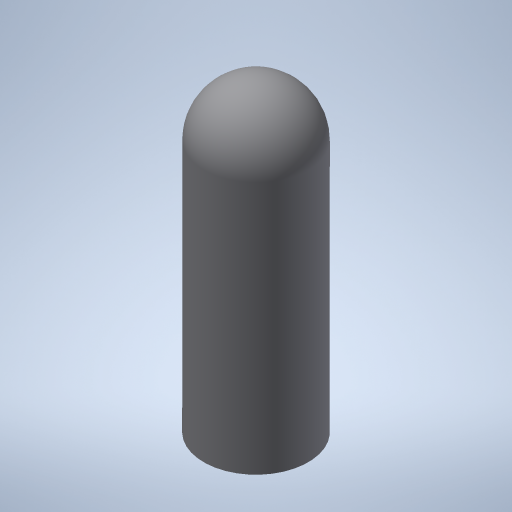
# Autodesk Inventor part: continuacion medio
Saved by Autodesk Inventor 2023 (Build 270158000, 158)
## iProperties
Created: 2022-10-21
Part Number: continuacion medio
Material: Generic
Document SubType Name: Modeling
Designer: Xiaba
Density: 1 g/cm^3
Appearance: Default
Author: Xiaba
Autodesk Inventor part; units mm, degrees
ref_plane "YZ Plane" through (0, 0, 0) normal (1, 0, 0) x (0, 1, 0)
ref_plane "XZ Plane" through (0, 0, 0) normal (0, 1, 0) x (-1, 0, 0)
ref_plane "XY Plane" through (0, 0, 0) normal (0, 0, 1) x (1, 0, 0)
sketch "Sketch1" plane through (0, 0, 0) normal (0, 1, 0) x (-1, 0, 0)
  circle A0 centre (0, 0) radius 0.875
  dimension "d0" = 1.75
  constraints: 1 centre point, 1 coincident
  measures "d0" diameter of A0
extrude "Extrusion1" add sketch "Sketch1" along normal blind 5.13
sketch "Sketch2" plane through (0, 0, 0) normal (1, 0, 0) x (0, 1, 0)
  line L0 (5.13, -0.875) -> (5.13, 0.875) projected
  arc A0 (5.13, 0.875) -> (5.13, -0.875) centre (5.111, 0) ccw
  line L1 (4.2358, 0) -> (4.2358, 0.875)
  line L2 (0, 0.875) -> (5.13, 0.875) projected
  line L3 (0, -0.875) -> (5.13, -0.875) projected
  arc A1 (4.2358, -0.875) -> (4.2358, 0.875) centre (4.236, 0) ccw
  line L4 (5.111, 0) -> (4.236, 0)
  line L5 (5.13, 0.875) -> (4.2358, 0.875)
  line L6 (4.2358, 0.875) -> (4.2358, -0.875)
  line L7 (4.2358, -0.875) -> (5.13, -0.875)
  line L8 (5.13, -0.875) -> (5.13, 0.875)
  line L9 (5.3365, 0) -> (4.983, 0)
  point P0 (0, 0)
  point P1 (5.13, 0)
  constraints: 14 end point, 6 point on circle, 3 point on line, 2 centre point, 2 horizontal, 2 parallel, 1 perpendicular, 1 vertical
revolve "Revolution1" cut sketch "Sketch2" angle 360 about axis through (0, 5.111, 0) along (0, -1, 0) picked at (5.0364, -0.5818) contours A0 A1 L9 L0 | L3 A1 A0
shell "Shell1" thickness 0.1 removed faces 1 at (0.2866, 0, -0.1766)
body "Solid1"
